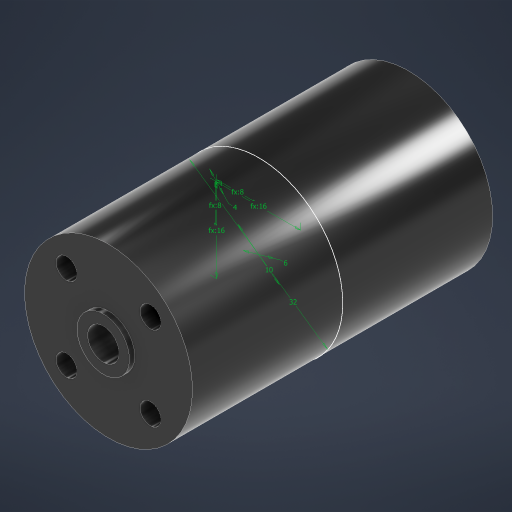
# Autodesk Inventor part: Generator
Saved by Autodesk Inventor 2023.2 (Build 272271000, 271)
## iProperties
Created: 2023-04-06
Part Number: Generator
Material: ABS-Kunststoff
Document SubType Name: Modeling
Designer: tadeus
Density: 1.06 g/cm^3
Appearance: Glatt - Weiß
Author: tadeus
Autodesk Inventor part; units mm, degrees
ref_plane "YZ Plane" through (0, 0, 0) normal (1, 0, 0) x (0, 1, 0)
ref_plane "XZ Plane" through (0, 0, 0) normal (0, 1, 0) x (-1, 0, 0)
ref_plane "XY Plane" through (0, 0, 0) normal (0, 0, 1) x (1, 0, 0)
sketch "Skizze1" plane through (0, 0, 0) normal (0, 0, 1) x (1, 0, 0)
  circle A0 centre (0, 0) radius 16
  circle A1 centre (-8, 8) radius 2
  line L0 (0, 16) -> (0, -16) construction
  line L1 (-16, 0) -> (16, 0) construction
  circle A2 centre (8, 8) radius 2
  circle A3 centre (-8, -8) radius 2
  circle A4 centre (8, -8) radius 2
  circle A5 centre (0, 0) radius 5
  circle A6 centre (0, 0) radius 3
  dimension "d0" = 32
  dimension "d1" = 4
  dimension "d2" = 8
  dimension "d3" = 8
  dimension "d6" = 16
  dimension "d9" = 16
  dimension "d16" = 10
  dimension "d19" = 6
  constraints: 7 centre point, 4 end point, 4 point on circle, 3 coincident, 3 vertical, 2 horizontal, 6 other
  measures "d0" diameter of A0
  measures "d1" diameter of A1
  measures "d2" distance from line of A1.centre L0
  measures "d3" distance from line of A1.centre L1
  measures "d6" distance of A1.centre A2.centre
  measures "d9" distance of A1.centre A3.centre
  measures "d16" diameter of A5
  measures "d19" diameter of A6
extrude "Extrusion1" add sketch "Skizze1" along normal mid plane 57.2 contours A0 | A1 | A2 | A3 | A4 | A5 | A6
extrude "Extrusion2" cut sketch "Skizze1" against normal blind 10 from surface at 28.6 contours A1 | A2 | A3 | A4
extrude "Extrusion3" add sketch "Skizze1" along normal blind 1 from surface at 28.6 contours A5 | A6
extrude "Extrusion4" cut sketch "Skizze1" along normal through all both and the other way through all contours A6
mirror "Spiegeln1" about plane through (0, 0, 0) normal (0, 0, 1) of "Extrusion2"
equation "\"d2\" = Montage"
equation "\"d3\" = Montage"
equation "\"d6\" = 2 * Montage"
equation "\"d9\" = 2 * Montage"
equation "\"Montage\" = 8"
